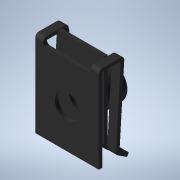
# Autodesk Inventor part: 8617.540_P3
Saved by Autodesk Inventor 2021 (Build 250183000, 183)
## iProperties
Created: 2026-08-04
Part Number: 8617.540_P3
Material: Generic
Catalog Web Link: www.3dfindit.com
Description: VX Teilmontageplatte - P3-VX Teilmontageplatte - P3
Vendor: RITTAL
Document SubType Name: Modeling
Designer: psAdmin
Manufacturer: RITTAL
Mass: 1.08452 g
Surface Area: 23.8149 cm^2
Volume: 1.08452 cm^3
Density: 1 g/cm^3
Appearance: PSOLRGB-176-176-176
Category: PARTsolutions
Company: RITTAL
Title: 8617.540_P3
Author: Cadenas PARTsolutions
Comments: VX Teilmontageplatte - P3
PSOL_IDENT_0: {$CADENAS_DATA/23d-libs/rittal/sys_zub/innenausbau/montageplatten/parts/teilmontageplatten_m51_p3.pr
PSOL_IDENT_1: j},181 {VTYP=3D},{NB=8617.540_P3},{LINA=8617.540_P3},{NN=VX Teilmontageplatte - P3},{DATE=16.02.2026
PSOL_IDENT_2: 20:13:30},{GEOMDATE=11.04.2025 11:24:24},{VERSION=},{LINEID=40},{WBVAR=},{WBNUMERIC=}  {NB=8617.540
PSOL_IDENT_3: _P3},{LINA=8617.540_P3},{KT=DUMMY},{BEST=8617.540},{INFO=PDF Katalog},{BEZ1=VX Teilmontageplatte},{B
PSOL_IDENT_4: EZ2=für neues Großschranksystem},{B=600},{BB=499},{H=800},{HH=699},{SB=600},{SH=800},{AB=600 x 800},
PSOL_IDENT_5: {VE=1},{VERS=4},{INFOPAGE=hb35_s707},{INFOPATH=hb35_s707_en.pdf},{CNSECLASS51=27-18-92-31},{CNSECLAS
PSOL_IDENT_6: S70=27-40-92-16},{CNSECLASS80=27-40-92-16},{CNSETIM40=EC000213},{BEZ3=},{DETAIL=1},{ADDGEO=1},{GEW=9
PSOL_IDENT_7: ,22},{CNSETIM80=EC000213},{CNSETIM90=EC000213},{CNSECLASS60=27-40-92-16},{UNSPSC=31-26-15-02}
NB: 8617.540_P3
NN: VX Teilmontageplatte - P3
NT: VX Teilmontageplatte - P3
NBSYN: $BEST._P3
LINA: 8617.540_P3
CATALOG: Rittal
BEST: 8617.540
INFO: PDF Katalog
BEZ1: VX Teilmontageplatte
BB: 499
HH: 699
SB: 600
SH: 800
CNSECLASS70: 27-40-92-16
CNSECLASS80: 27-40-92-16
GEW: 9,22
CNSETIM80: EC000213
CNSETIM90: EC000213
CNSECLASS60: 27-40-92-16
UNSPSC: 31-26-15-02
SUPPLIER: RITTAL
ARTICLENO: 8617.540_P3
BOMINFO: 8617.540_P3
CREATOR: CADENAS GmbH
Autodesk Inventor part; units mm, degrees
sketch "Sketch_1" plane through (0, 0, 0) normal (1, 0, 0) x (0, 0, -1)
  line L0 (0, 12.3912) -> (0, -11.05)
  line L1 (0, -11.05) -> (1, -11.05)
  line L2 (1, -11.05) -> (1, 12.4)
  line L3 (1, 12.4) -> (5.6693, 12.4)
  arc A0 (6.1684, 11.8695) -> (5.6693, 12.4) centre (5.6693, 11.9) ccw
  line L4 (6.1684, 11.8695) -> (4.8747, -9.2828)
  arc A1 (4.8747, -9.2828) -> (5.3282, -10.1825) centre (5.8728, -9.3439) ccw
  line L5 (5.3282, -10.1825) -> (7.9554, -11.8887)
  line L6 (7.9554, -11.8887) -> (8.5, -11.05)
  line L7 (8.5, -11.05) -> (6.1173, -9.5027)
  arc A2 (5.8906, -9.0528) -> (6.1173, -9.5027) centre (6.3897, -9.0834) ccw
  line L8 (5.8906, -9.0528) -> (7.1957, 12.2848)
  arc A3 (7.1957, 12.2848) -> (6.2063, 13.3458) centre (6.1975, 12.3459) ccw
  line L9 (6.2063, 13.3458) -> (1.0087, 13.3912)
  arc A4 (1.0087, 13.3912) -> (0, 12.3912) centre (1, 12.3912) ccw
  constraints: 20 end point, 10 point on circle, 5 centre point
extrude "Extrusion1" add sketch "Sketch_1" along normal mid plane 18
sketch "Sketch_2" plane through (0, 0, 0) normal (0, 0, 1) x (1, 0, 0)
  line L0 (-6.75, 16.5) -> (-6.75, 12.5)
  arc A0 (-6.75, 12.5) -> (-5.75, 11.5) centre (-5.75, 12.5) ccw
  line L1 (-5.75, 11.5) -> (5.75, 11.5)
  arc A1 (5.75, 11.5) -> (6.75, 12.5) centre (5.75, 12.5) ccw
  line L2 (6.75, 12.5) -> (6.75, 16.5)
  line L3 (6.75, 16.5) -> (-6.75, 16.5)
  constraints: 8 end point, 4 point on circle, 2 centre point
extrude "Extrusion2" cut sketch "Sketch_2" against normal blind 8
sketch "Sketch_3" plane through (0, 0, -1) normal (0, 0, 1) x (1, 0, 0)
  line L0 (-6.5, -12) -> (6.5, -12)
  line L1 (6.5, -12) -> (6.5, 13)
  line L2 (6.5, 13) -> (-6.5, 13)
  line L3 (-6.5, 13) -> (-6.5, -12)
  constraints: 8 end point
extrude "Extrusion3" cut sketch "Sketch_3" against normal blind 8
sketch "Sketch_4" plane through (0, 0, 0) normal (1, 0, 0) x (0, 0, -1)
  arc A0 (4, -7.9626) -> (5.1384, -10.0593) centre (6.5, -7.9626) ccw
  line L0 (5.1384, -10.0593) -> (7.9554, -11.8887)
  line L1 (7.9554, -11.8887) -> (8.5, -11.05)
  line L2 (8.5, -11.05) -> (5.4554, -9.0728)
  arc A1 (5, -8.2341) -> (5.4554, -9.0728) centre (6, -8.2341) ccw
  line L3 (5, -8.2341) -> (5, 13.4)
  line L4 (5, 13.4) -> (4, 13.4)
  line L5 (4, 13.4) -> (4, -7.9626)
  constraints: 12 end point, 4 point on circle, 2 centre point
extrude "Extrusion4" add sketch "Sketch_4" along normal mid plane 13
sketch "Sketch_5" plane through (0, 0, 0) normal (1, 0, 0) x (0, 0, -1)
  line L0 (13, 0) -> (4, 0)
  line L1 (4, 0) -> (4, 5.7)
  line L2 (4, 5.7) -> (5, 5.7)
  arc A0 (5, 5.7) -> (6, 4.7) centre (6, 5.7) ccw
  line L3 (6, 4.7) -> (12, 4.7)
  arc A1 (13, 3.7) -> (12, 4.7) centre (12, 3.7) ccw
  line L4 (13, 3.7) -> (13, 0)
  line L5 (13, 0) -> (4, 0)
  constraints: 12 end point, 4 point on circle, 2 centre point
revolve "Revolution1" add sketch "Sketch_5" angle 360 about axis through (0, 0, -13) along (0, 0, -1)
sketch "Sketch6" plane through (0, 0, -13) normal (0, 0, -1) x (-1, 0, 0)
  point P0 (0, 0)
hole "Hole1" at (0, 0, -13) direction (0, 0, 1) diameter 7 depth 14
ref_plane "P3_XY" through (0, 0, 0) normal (0, 0, -1) x (1, 0, 0)
ref_plane "P3_YZ" through (0, 0, 0) normal (1, 0, 0) x (0, -1, 0)
ref_plane "P3_ZX" through (0, 0, 0) normal (0, -1, 0) x (0, 0, -1)
body "Solid1"
